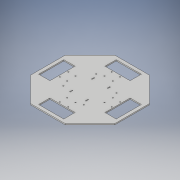
# Autodesk Inventor part: Base
Saved by Autodesk Inventor 2019 (Build 230136000, 136)
## iProperties
Created: 2019-03-08
Part Number: Base
Material: Generic
Document SubType Name: Modeling
Designer: jonas
Density: 1 g/cm^3
Appearance: Default
Author: jonas
Autodesk Inventor part; units mm, degrees
ref_plane "YZ Plane" through (0, 0, 0) normal (1, 0, 0) x (0, 1, 0)
ref_plane "XZ Plane" through (0, 0, 0) normal (0, 1, 0) x (-1, 0, 0)
ref_plane "XY Plane" through (0, 0, 0) normal (0, 0, 1) x (1, 0, 0)
sketch "Sketch2" plane through (0, 0, 0) normal (0, 1, 0) x (-1, 0, 0)
  line L0 (-54, -130.3675) -> (-130.3675, -54)
  line L1 (-130.3675, -54) -> (-130.3675, 54)
  line L2 (-130.3675, 54) -> (-54, 130.3675)
  line L3 (-54, 130.3675) -> (54, 130.3675)
  line L4 (54, 130.3675) -> (130.3675, 54)
  line L5 (130.3675, 54) -> (130.3675, -54)
  line L6 (130.3675, -54) -> (54, -130.3675)
  line L7 (54, -130.3675) -> (-54, -130.3675)
  line L8 (264.6809, 0) -> (-264.6809, 0) projected
  line L9 (-39, -120.3675) -> (39, -120.3675)
  line L10 (39, -120.3675) -> (39, -85.3675)
  line L11 (39, -85.3675) -> (-39, -85.3675)
  line L12 (-39, -85.3675) -> (-39, -120.3675)
  line L13 (85.3675, -39) -> (120.3675, -39)
  line L14 (85.3675, 39) -> (85.3675, -39)
  line L15 (120.3675, -39) -> (120.3675, 39)
  line L16 (120.3675, 39) -> (85.3675, 39)
  line L17 (39, 85.3675) -> (39, 120.3675)
  line L18 (-39, 85.3675) -> (39, 85.3675)
  line L19 (39, 120.3675) -> (-39, 120.3675)
  line L20 (-39, 120.3675) -> (-39, 85.3675)
  line L21 (-85.3675, 39) -> (-120.3675, 39)
  line L22 (-85.3675, -39) -> (-85.3675, 39)
  line L23 (-120.3675, 39) -> (-120.3675, -39)
  line L24 (-120.3675, -39) -> (-85.3675, -39)
  circle A0 centre (-13.125, -80.3675) radius 1.6
  line L25 (0, -182.5145) -> (0, 182.5145) projected
  circle A1 centre (-13.125, -58.0175) radius 1.6
  circle A2 centre (13.125, -80.3675) radius 1.6
  circle A3 centre (13.125, -58.0175) radius 1.6
  circle A4 centre (80.3675, -13.125) radius 1.6
  circle A5 centre (80.3675, 13.125) radius 1.6
  circle A6 centre (58.0175, -13.125) radius 1.6
  circle A7 centre (58.0175, 13.125) radius 1.6
  circle A8 centre (13.125, 80.3675) radius 1.6
  circle A9 centre (-13.125, 80.3675) radius 1.6
  circle A10 centre (13.125, 58.0175) radius 1.6
  circle A11 centre (-13.125, 58.0175) radius 1.6
  circle A12 centre (-80.3675, 13.125) radius 1.6
  circle A13 centre (-80.3675, -13.125) radius 1.6
  circle A14 centre (-58.0175, 13.125) radius 1.6
  circle A15 centre (-58.0175, -13.125) radius 1.6
  line L26 (-23.5, -38) -> (-25.5, -38)
  line L27 (-25.5, -38) -> (-25.5, -30)
  line L28 (-25.5, -30) -> (-23.5, -30)
  line L29 (-23.5, -30) -> (-23.5, -38)
  line L30 (-264.6809, 0) -> (264.6809, 0)
  line L31 (23.5, -38) -> (25.5, -38)
  line L32 (25.5, -38) -> (25.5, -30)
  line L33 (25.5, -30) -> (23.5, -30)
  line L34 (23.5, -30) -> (23.5, -38)
  line L35 (-23.5, 38) -> (-25.5, 38)
  line L36 (-25.5, 38) -> (-25.5, 30)
  line L37 (-25.5, 30) -> (-23.5, 30)
  line L38 (-23.5, 30) -> (-23.5, 38)
  line L39 (25.5, 38) -> (25.5, 30)
  line L40 (25.5, 30) -> (23.5, 30)
  line L41 (23.5, 30) -> (23.5, 38)
  line L42 (23.5, 38) -> (25.5, 38)
  circle A16 centre (-31.5917, 50.9465) radius 1.6
  circle A17 centre (-50.9465, -31.5917) radius 1.6
  circle A18 centre (31.5917, -50.9465) radius 1.6
  circle A19 centre (50.9465, 31.5917) radius 1.6
  point P0 (0, 0)
  point P1 (0, 0)
  point P2 (0, 0)
  point P3 (0, 0)
  point P4 (0, 0)
  dimension "d5" = 10
  dimension "d6" = 35
  dimension "d7" = 15
  dimension "d8" = 15
  dimension "d11" = 360
  dimension "d13" = 78
  dimension "d14" = 13.125
  dimension "d16" = 5
  dimension "d18" = 22.35
  dimension "d21" = 360
  dimension "d23" = 23.5
  dimension "d24" = 2
  dimension "d25" = 8
  dimension "d26" = 30
  dimension "d28" = 3.2
  dimension "d29" = 3.2
  dimension "d32" = 360
  constraints: 82 end point, 20 centre point, 16 symmetric about line, 4 parallel, 3 coincident, 3 perpendicular, 2 horizontal, 1 equal radius, 96 other
  measures "d5" distance between parallel lines of L9 L7
  measures "d6" distance between parallel lines of L11 L9
  measures "d7" distance from line of L0.start L12
  measures "d8" distance from line of L6.end L10
  measures "d13" distance between parallel lines of L12 L10
  measures "d14" distance from line of L25 A0.centre
  measures "d16" distance from line of A0.centre L11
  measures "d18" distance of A1.centre A0.centre
  measures "d23" distance between parallel lines of L29 L25
  measures "d24" distance between parallel lines of L27 L29
  measures "d25" distance between parallel lines of L28 L26
  measures "d26" distance between parallel lines of L28 L8
  measures "d28" diameter of A16
  measures "d29" diameter of A3
extrude "Extrusion1" add sketch "Sketch2" along normal blind 3.5 contours L0 L1 L8 L23 L24 L22 L25 L11 L12 L9 L7 | L25 L9 L10 L11 L8 L14 L13 L15 L5 L6 L7 | L1 L2 L3 L25 L19 L20 L18 L8 L22 L21 L23 | L8 L15 L16 L14 L25 L18 L17 L19 L3 L4 L5
equation "\"d8\" = d7"
body "Solid1"
